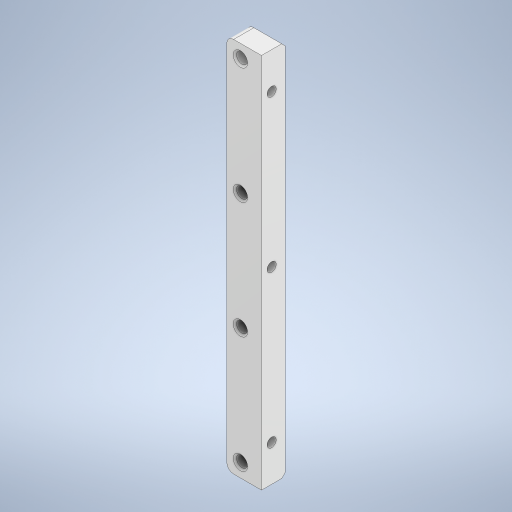
# Autodesk Inventor part: Door Bar Front Panel Mount
Saved by Autodesk Inventor 2024 (Build 280153000, 153)
## iProperties
Created: 2024-12-01
Part Number: Door Bar Front Panel Mount
Material: ABS Plastic
Document SubType Name: Modeling
Designer: Ishaan
Density: 1.06 g/cm^3
Appearance: Smooth - White
Author: Ishaan
Autodesk Inventor part; units mm, degrees
ref_plane "YZ Plane" through (0, 0, 0) normal (1, 0, 0) x (0, 1, 0)
ref_plane "XZ Plane" through (0, 0, 0) normal (0, 1, 0) x (-1, 0, 0)
ref_plane "XY Plane" through (0, 0, 0) normal (0, 0, 1) x (1, 0, 0)
sketch "Sketch1" plane through (0, 0, 0) normal (0, 0, 1) x (1, 0, 0)
  line L0 (10.25, -111.5) -> (-10.25, -111.5)
  line L1 (-10.25, -111.5) -> (-10.25, 111.5)
  line L2 (-10.25, 111.5) -> (10.25, 111.5)
  line L3 (10.25, 111.5) -> (10.25, -111.5)
  line L4 (10.25, -111.5) -> (-10.25, 111.5) construction
  line L5 (-10.25, -111.5) -> (10.25, 111.5) construction
  line L6 (-2.25, 103.5) -> (-2.25, -103.5) construction
  point P0 (0, 0)
  point P1 (-2.25, 34.5)
  point P2 (-2.25, -34.5)
  point P3 (-2.25, 0)
  dimension "d0" = 20.5
  dimension "d4" = 69
  dimension "d9" = 8
  dimension "d10" = 8
  constraints: 14 end point, 3 midpoint, 2 coincident, 2 parallel, 2 vertical, 1 horizontal, 1 horizontal alignment, 1 perpendicular, 3 other
  measures "d0" distance of L1.end L2.end
  measures "d4" distance of point (-2.25, 103.5) point (-2.25, 34.5)
  measures "d9" distance from line of L6.start L2
  measures "d10" distance from line of L6.start L1
extrude "Extrusion1" add sketch "Sketch1" against normal blind 14
fillet "Fillet1" radius 4 2 edges at (-10.25, 111.5, -7) (-10.25, -111.5, -7)
chamfer "Chamfer1" distance 2 angle 45 5 edges at (2, 111.5, -14) (-9.0784, 110.3284, -14) (-10.25, 0, -14) (-9.0784, -110.3284, -14) (2, -111.5, -14)
hole "Hole1" at (-2.25, 103.5, 0) at (-2.25, 34.5, 0) at (-2.25, -34.5, 0) at (-2.25, -103.5, 0) direction (0, 0, -1) diameter 6.5 end through all
sketch "Sketch2" plane through (-10.25, -107.5, 0) normal (-1, 0, 0) x (0, 0, 1)
  line L0 (-6, 197.5) -> (-6, 17.5) construction
  line L1 (0, 215) -> (0, 0) projected
  point P0 (0, 107.5)
  point P1 (0, 107.5)
  point P2 (-6, 107.5)
  point P3 (-6, 107.5)
  dimension "d24" = 180
  dimension "d25" = 6
  constraints: 3 coincident, 2 end point, 2 midpoint, 1 horizontal alignment, 1 vertical
  measures "d24" distance of L0.start L0.end
  measures "d25" distance between parallel lines of L1 L0
hole "Hole2" at (-10.25, 90, -6) at (-10.25, 0, -6) at (-10.25, -90, -6) direction (1, 0, 0) diameter 5.4 end through all counterbore diameter 9.5 counterbore depth 6.5
chamfer "Chamfer2" distance 1 angle 45 4 edges at (-2.25, -100.25, 0) (-2.25, -31.25, 0) (-2.25, 37.75, 0) (-2.25, 106.75, 0)
equation "\"d10\" = d9"
body "Solid1"
